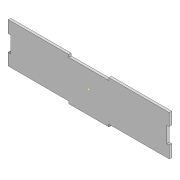
# Autodesk Inventor part: 본체 겉면 레이저 옆판 수정
Saved by Autodesk Inventor 2020 (Build 240168000, 168)
## iProperties
Created: 2022-08-25
Part Number: 본체 겉면 레이저 옆판 수정
Material: 일반
Document SubType Name: Modeling
Designer: 박연호
Density: 1 g/cm^3
Appearance: 기본값
Author: 박연호
Autodesk Inventor part; units mm, degrees
ref_plane "YZ Plane" through (0, 0, 0) normal (1, 0, 0) x (0, 1, 0)
ref_plane "XZ Plane" through (0, 0, 0) normal (0, 1, 0) x (-1, 0, 0)
ref_plane "XY Plane" through (0, 0, 0) normal (0, 0, 1) x (1, 0, 0)
sketch "스케치1" plane through (0, 0, 0) normal (0, 0, 1) x (1, 0, 0)
  line L0 (-100, -25) -> (100, -25)
  line L1 (100, -25) -> (100, 25)
  line L2 (100, 25) -> (-100, 25)
  line L3 (-100, 25) -> (-100, -25)
  line L4 (-100, -25) -> (100, 25) construction
  line L5 (100, -25) -> (-100, 25) construction
  line L6 (-25, 22) -> (25, 22)
  line L7 (25, 22) -> (25, 28)
  line L8 (25, 28) -> (-25, 28)
  line L9 (-25, 28) -> (-25, 22)
  line L10 (-25, 22) -> (25, 28) construction
  line L11 (25, 22) -> (-25, 28) construction
  line L12 (-103, -10) -> (-97, -10)
  line L13 (-97, -10) -> (-97, 10)
  line L14 (-97, 10) -> (-103, 10)
  line L15 (-103, 10) -> (-103, -10)
  line L16 (-103, -10) -> (-97, 10) construction
  line L17 (-97, -10) -> (-103, 10) construction
  line L18 (97, -10) -> (103, -10)
  line L19 (103, -10) -> (103, 10)
  line L20 (103, 10) -> (97, 10)
  line L21 (97, 10) -> (97, -10)
  line L22 (97, -10) -> (103, 10) construction
  line L23 (103, -10) -> (97, 10) construction
  point P0 (0, 0)
  point P1 (0, 25)
  point P2 (-100, 0)
  point P3 (100, 0)
  point P4 (-100, -10)
  point P5 (100, -10)
  point P6 (100, 10)
  point P7 (25, 25)
  point P8 (-25, 25)
  point P9 (-100, 10)
  dimension "d0" = 50
  dimension "d1" = 200
  dimension "d2" = 50
  dimension "d3" = 3
  dimension "d4" = 20
  dimension "d5" = 20
  dimension "d6" = 3
  dimension "d7" = 3
  constraints: 48 end point, 11 midpoint, 8 parallel, 4 horizontal, 4 perpendicular
  measures "d0" distance of L2.end L0.start
  measures "d1" distance of L1.end L2.end
  measures "d2" distance of L8.end L7.end
  measures "d3" distance between parallel lines of L6 L2
  measures "d4" distance of L13.end L12.end
  measures "d5" distance of L19.end L18.end
  measures "d6" distance between parallel lines of L21 L1
  measures "d7" distance between parallel lines of L3 L13
extrude "돌출1" add sketch "스케치1" along normal blind 3 contours L3 L12 L13 L14 L2 L9 L6 L7 L1 L20 L21 L18 L0
sketch "스케치2" plane through (0, 0, 3) normal (0, 0, 1) x (1, 0, 0)
  line L0 (-25, -22) -> (25, -22)
  line L1 (25, -22) -> (25, -28)
  line L2 (25, -28) -> (-25, -28)
  line L3 (-25, -28) -> (-25, -22)
  line L4 (-100, -25) -> (100, -25) projected
  line L5 (-25, -22) -> (25, -28) construction
  line L6 (25, -22) -> (-25, -28) construction
  point P0 (0, 0)
  point P1 (0, -25)
  point P2 (25, -25)
  point P3 (-25, -25)
  dimension "d10" = 50
  dimension "d11" = 3
  constraints: 12 end point, 3 midpoint, 2 parallel, 1 horizontal, 1 perpendicular
  measures "d10" distance of L1.end L2.end
  measures "d11" distance between parallel lines of L2 L4
extrude "돌출2" add sketch "스케치2" against normal blind 3 contours L4 L1 L2 L3
sketch "스케치3" plane through (0, 0, 3) normal (0, 0, 1) x (1, 0, 0)
  point P0 (0, 0)
